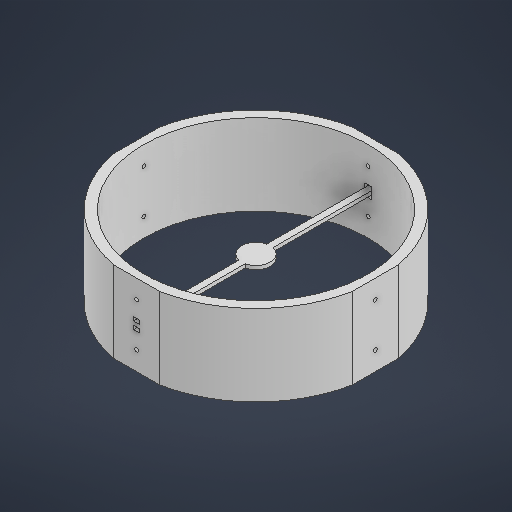
# Autodesk Inventor part: 001-001
Saved by Autodesk Inventor 2026 (Build 300175000, 175)
## iProperties
Created: 2026-04-19
Part Number: 001-001
Material: Ogólny
Document SubType Name: Modeling
Designer: Patryk Lombardo
Density: 1 g/cm^3
Appearance: Domyślna
Author: Patryk Lombardo
Autodesk Inventor part; units mm, degrees
ref_plane "YZ Plane" through (0, 0, 0) normal (1, 0, 0) x (0, 1, 0)
ref_plane "XZ Plane" through (0, 0, 0) normal (0, 1, 0) x (-1, 0, 0)
ref_plane "XY Plane" through (0, 0, 0) normal (0, 0, 1) x (1, 0, 0)
sketch "okrąg" plane through (0, 0, 0) normal (0, 1, 0) x (-1, 0, 0)
  circle A0 centre (0, 0) radius 90
  circle A1 centre (0, 0) radius 97.5
  line L0 (0, 0) -> (0, -95.75) construction
  line L1 (-18.3899, -95.75) -> (18.3899, -95.75)
  line L2 (0, 0) -> (95.75, 0) construction
  line L3 (95.75, -18.3899) -> (95.75, 18.3899)
  line L4 (0, 0) -> (0, 95.75) construction
  line L5 (18.3899, 95.75) -> (-18.3899, 95.75)
  line L6 (0, 0) -> (-95.75, 0) construction
  line L7 (-95.75, 18.3899) -> (-95.75, -18.3899)
  point P0 (-95.75, 18.3899)
  point P1 (-95.75, -18.3899)
  point P2 (-18.3899, -95.75)
  point P3 (95.75, -18.3899)
  point P4 (95.75, 18.3899)
  point P5 (18.3899, 95.75)
  point P6 (-18.3899, 95.75)
  dimension "d1" = 195
  dimension "d0" = 180
  dimension "d2" = 95.75
  dimension "d5" = 360
  constraints: 16 end point, 2 coincident, 1 centre point, 1 horizontal, 1 midpoint, 1 vertical, 28 other
  measures "d0" diameter of A0
  measures "d2" distance of L0.start L0.end
extrude "Wyciągnięcie proste1" add sketch "okrąg" along normal mid plane 65 contours L3 A1 L1 L7 L5
sketch "podpora" plane through (0, 0, 0) normal (0, 1, 0) x (-1, 0, 0)
  circle A0 centre (0, 0) radius 90
  line L0 (2.5, 0) -> (-2.5, 0) construction
  line L1 (-2.5, -90) -> (-2.5, 90)
  line L2 (2.5, -90) -> (2.5, 90)
  circle A1 centre (0, 0) radius 11.5
  point P0 (-2.5, -11.225)
  point P1 (-2.5, -89.9653)
  point P2 (2.5, -89.9653)
  point P3 (2.5, -11.225)
  point P4 (2.5, 11.225)
  point P5 (2.5, 89.9653)
  point P6 (-2.5, 89.9653)
  point P7 (-2.5, 11.225)
  dimension "d12" = 180
  dimension "d13" = 5
  dimension "d14" = 180
  dimension "d15" = 180
  dimension "d16" = 23
  constraints: 6 end point, 3 midpoint, 2 centre point, 2 coincident, 2 vertical, 1 horizontal
  measures "d12" diameter of A0
  measures "d13" distance of L0.start L0.end
  measures "d14" distance of L1.start L1.end
  measures "d15" distance of L2.start L2.end
  measures "d16" diameter of A1
extrude "Wyciągnięcie proste2" add sketch "podpora" along normal mid plane 3 contours L2 A1 L1 A0 | A0 L1 A1 L2 | A1 L2 | L2 A1 L1 | L1 A1
sketch "Szkic5" plane through (-18.3899, 32.5, 95.75) normal (0, 0, 1) x (1, 0, 0)
  line L0 (0, 0) -> (18.3899, 0) construction
  line L1 (18.3899, 0) -> (18.3899, -15) construction
  line L2 (18.3899, -15) -> (18.3899, -50) construction
  circle A0 centre (18.3899, -15) radius 1.5
  circle A1 centre (18.3899, -50) radius 1.5
  point P0 (18.3899, -32.5)
  dimension "d28" = 18.3899
  dimension "d32" = 32.5
  dimension "d33" = 32.5
  dimension "d34" = 15
  dimension "d35" = 35
  dimension "d36" = 3
  dimension "d37" = 3
  constraints: 6 end point, 2 centre point, 2 coincident, 1 horizontal, 1 point on line, 1 vertical
  measures "d28" distance of L0.start L0.end
  measures "d32" distance from line of point (18.39, -32.5) L0
  measures "d33" distance of point (18.39, -32.5) L0.end
  measures "d34" distance of L0.end L1.end
  measures "d35" distance of L1.end L2.end
  measures "d36" diameter of A0
  measures "d37" diameter of A1
extrude "Wyciągnięcie proste4" cut sketch "Szkic5" against normal through all
sketch "Szkic6" plane through (-95.75, -32.5, 18.3899) normal (-1, 0, 0) x (0, 0, 1)
  line L0 (-18.3899, 32.5) -> (-18.3899, 50) construction
  line L1 (-18.3899, 32.5) -> (-18.3899, 15) construction
  circle A0 centre (-18.3899, 15) radius 1.5
  circle A1 centre (-18.3899, 50) radius 1.5
  dimension "d40" = 17.5
  dimension "d41" = 17.5
  dimension "d42" = 3
  dimension "d43" = 3
  constraints: 4 end point, 2 centre point, 2 coincident, 2 vertical
  measures "d40" distance of L0.start L0.end
  measures "d41" distance of L0.start L1.end
  measures "d42" diameter of A1
  measures "d43" diameter of A0
extrude "Wyciągnięcie proste5" cut sketch "Szkic6" against normal through all
sketch "Szkic7" plane through (18.3899, 32.5, -95.75) normal (0, 0, -1) x (-1, 0, 0)
  line L0 (18.3899, -31) -> (18.3899, -34) construction
  line L1 (15.8899, -31) -> (20.8899, -31)
  line L2 (20.8899, -31) -> (20.8899, -28)
  line L3 (20.8899, -28) -> (15.8899, -28)
  line L4 (15.8899, -28) -> (15.8899, -31)
  line L5 (15.8899, -34) -> (20.8899, -34)
  line L6 (20.8899, -34) -> (20.8899, -37)
  line L7 (20.8899, -37) -> (15.8899, -37)
  line L8 (15.8899, -37) -> (15.8899, -34)
  point P0 (18.3899, -32.5)
  dimension "d46" = 3
  dimension "d47" = 5
  dimension "d48" = 3
  dimension "d49" = 3
  dimension "d50" = 5
  constraints: 18 end point, 4 horizontal, 3 midpoint, 3 vertical, 2 perpendicular
  measures "d46" distance of L0.start L0.end
  measures "d47" distance of L1.start L1.end
  measures "d48" distance of L1.end L2.end
  measures "d49" distance of L5.end L6.end
  measures "d50" distance of L5.start L5.end
extrude "Wyciągnięcie proste6" cut sketch "Szkic7" against normal through all
equation "\"d12\" = d0"
equation "\"d14\" = d0"
equation "\"d15\" = d0"
